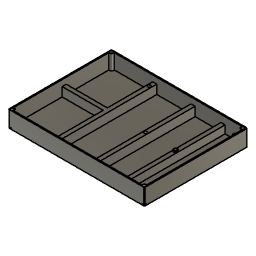
Housing_Base (Autodesk Fusion 360 design; units mm, degrees)
Autodesk Fusion 360 part; units mm, degrees
sketch "Sketch1" plane through (0, 0, 0) normal (0, 0, 1) x (1, 0, 0)
  line L0 (267, 172) -> (40, 172)
  line L1 (40, 172) -> (40, 0)
  line L2 (267, 0) -> (267, 172)
  circle A0 centre (114.1412, 160.8678) radius 2.55
  circle A1 centre (114.1412, 7.8678) radius 2.55
  circle A2 centre (257.1412, 7.8678) radius 2.55
  circle A3 centre (228.1412, 90.8678) radius 2.55
  circle A4 centre (178.1412, 90.8678) radius 2.55
  circle A5 centre (257.1412, 161.8678) radius 2.55
  line L3 (231.5912, 2) -> (231.5912, 170)
  line L4 (231.5912, 2) -> (231.5912, 170)
  line L5 (267, 172) -> (40, 172)
  line L6 (267, 2) -> (267, 172)
  line L7 (40, 0) -> (267, 0)
  line L8 (265, 6.0151) -> (265, 165.4022)
  line L9 (260.0451, 170) -> (231.5912, 170)
  arc A6 (42, 165.4407) -> (46.5116, 170) centre (43.2595, 168.7062) ccw
  arc A7 (42, 165.4407) -> (46.5116, 170) centre (43.2595, 168.7062) ccw
  arc A8 (46.8079, 2) -> (42, 6.1449) centre (43.4407, 2.9551) ccw
  line L10 (224.6912, 2) -> (224.6912, 87.4178)
  line L11 (224.6912, 94.3178) -> (224.6912, 170)
  line L12 (42, 165.4407) -> (42, 94.3178)
  line L13 (42, 87.4178) -> (42, 6.1449)
  line L14 (110.6912, 170) -> (46.5116, 170)
  line L15 (42, 94.3178) -> (110.6912, 94.3178)
  line L16 (117.5912, 2) -> (117.5912, 87.4178)
  line L17 (117.5912, 94.3178) -> (117.5912, 170)
  line L18 (109.8811, 164.7657) -> (109.8811, 94.3178) construction
  line L19 (109.8811, 87.4178) -> (109.8811, 4.2996) construction
  line L20 (42, 87.4178) -> (110.6912, 87.4178)
  line L21 (110.6912, 2) -> (110.6912, 87.4178)
  line L22 (110.6912, 94.3178) -> (110.6912, 170)
  line L23 (46.8079, 2) -> (110.6912, 2)
  arc A9 (260.0451, 170) -> (265, 165.4022) centre (263.1412, 168.3678) ccw
  arc A10 (265, 6.0151) -> (260.8505, 2) centre (263.9632, 2.9349) ccw
  line L24 (231.5912, 2) -> (260.8505, 2)
  circle A11 centre (257.1412, 7.8678) radius 4
  circle A12 centre (257.1412, 161.8678) radius 4
  circle A13 centre (228.1412, 90.8678) radius 3.45
  line L25 (117.5912, 94.3178) -> (117.5912, 87.4178)
  line L26 (224.6912, 170) -> (231.5912, 170)
  line L27 (224.6912, 2) -> (231.5912, 2)
  line L28 (224.6912, 94.3178) -> (224.6912, 87.4178)
  line L29 (40, 0) -> (267, 0)
  line L30 (267, 0) -> (267, 172)
  line L31 (267, 172) -> (40, 172)
  line L32 (40, 172) -> (40, 0)
  line L33 (174.6912, 2) -> (174.6912, 170)
  line L34 (181.5912, 2) -> (181.5912, 170)
  line L35 (224.6912, 170) -> (181.5912, 170)
  line L36 (174.6912, 170) -> (117.5912, 170)
  line L37 (117.5912, 2) -> (174.6912, 2)
  line L38 (181.5912, 2) -> (224.6912, 2)
  line L39 (42, 94.3178) -> (42, 87.4178)
  line L40 (110.6912, 170) -> (117.5912, 170)
  line L41 (110.6912, 2) -> (117.5912, 2)
  line L42 (174.6912, 2) -> (181.5912, 2)
  line L43 (174.6912, 170) -> (181.5912, 170)
  circle A14 centre (263.1412, 168.3678) radius 2.55
  circle A15 centre (263.9632, 2.9349) radius 2.55
  line L44 (263.9632, 2.9349) -> (260.7497, 2.9349)
  circle A16 centre (43.2595, 168.7062) radius 2.55
  circle A17 centre (43.4407, 2.9551) radius 2.55
  dimension "d7" = 5.1
  dimension "d8" = 5.1
  dimension "d9" = 5.1
  dimension "d10" = 5.1
  dimension "d11" = 5.1
  dimension "d12" = 5.1
  dimension "d20" = 7
  dimension "d21" = 7
  dimension "d26" = 7
  dimension "d28" = 6.5
  dimension "d29" = 8
  dimension "d30" = 8
  dimension "d37" = 6.9
  dimension "d51" = 6.9
  dimension "d90" = 5.1
  dimension "d91" = 5.1
  dimension "d92" = 5.1
  dimension "d93" = 5.1
  constraint vertical L18
  constraint coincident L3.start L23
  constraint coincident L1 L7.start
  constraint coincident L11.end L9
  constraint collinear L9 L35
  constraint collinear L23 L24
  constraint concentric A6 A7
  constraint perpendicular L10 L20
  constraint coincident L13.start L12
  constraint collinear L10 L11
  constraint collinear L12 L13
  constraint perpendicular L16 L35
  constraint coincident L16.start L23
  constraint collinear L14 L35
  constraint coincident L15.end L21
  constraint coincident L17.start L16
  constraint coincident L16.end L20
  constraint collinear L16 L17
  constraint coincident L15 L18.end
  constraint coincident L19.start L20
  constraint collinear L18 L19
  constraint collinear L21 L22
  constraint collinear L23 L37
  constraint concentric A2 A11
  constraint concentric A5 A12
  constraint concentric A3 A13
  constraint perpendicular L4 L26
  constraint perpendicular L4 L27
  constraint horizontal L29
  constraint vertical L30
  constraint horizontal L31
  constraint vertical L32
  constraint coincident L33.end L35
  constraint perpendicular L33 L35
  constraint collinear L35 L36
  constraint collinear L37 L38
  constraint perpendicular L20 L39
  constraint perpendicular L16 L41
  constraint concentric A9 A14
  constraint concentric A10 A15
  constraint coincident A10.centre A15.centre
  constraint horizontal L44
  constraint concentric A6 A16
  constraint concentric A8 A17
  measures "d7" diameter of A0
  measures "d8" diameter of A1
  measures "d9" diameter of A2
  measures "d10" diameter of A5
  measures "d11" diameter of A4
  measures "d12" diameter of A3
  measures "d20" diameter of A6
  measures "d21" diameter of A8
  measures "d26" diameter of A9
  measures "d28" diameter of A10
  measures "d29" diameter of A11
  measures "d30" diameter of A12
  measures "d37" diameter of A13
  measures "d90" diameter of A14
  measures "d91" diameter of A15
  measures "d92" diameter of A16
  measures "d93" diameter of A17
extrude "Extrude4" add sketch "Sketch1" along normal blind 27 contours L0 L1 L2 L5 L6 L7 L29 L30 L31 L32 | A14 | A15 | A16 | A17 makes body 1
extrude "Extrude5" add sketch "Sketch1" along normal blind 15 separate body contours L3 L4 L10 A13 L27 L28 | L3 L4 L11 A13 L26 L28 makes body 2 at (224.6912, 31.6226, 5)
extrude "Extrude9" add sketch "Sketch1" along normal blind 2 separate body contours A2 makes body 3
extrude "Extrude11" add sketch "Sketch1" along normal blind 2 separate body contours A5 makes body 4
extrude "Extrude12" add sketch "Sketch1" along normal blind 2 separate body contours A0 | A1 | A3 | A4 makes body 5 at (116.6123, 161.4971, 1.3333) makes body 6 at (230.6406, 90.3626, 1.3333) makes body 7 at (116.0946, 9.5069, 1.3333) makes body 8 at (180.6406, 90.3626, 1.3333)
extrude "Extrude13" add sketch "Sketch1" along normal blind 17 contours A13 bodies 2 6
extrude "Extrude14" add sketch "Sketch1" along normal blind 17 contours L33 L34 L42 L43 | L15 L16 L17 L20 L21 L22 L25 L39 L40 L41 | A11 | A12 bodies 1 3 4 5 7 8
extrude "Extrude15" add sketch "Sketch1" along normal blind 2 contours L3 L4 L8 L9 A9 A10 L24 | L10 L11 L28 L34 L35 L38 | L16 L17 L25 L33 L36 L37 | A8 L13 L20 L21 L23 | A6 A7 L12 L14 L15 L22 bodies 1 2 3 4
extrude "Extrude16" cut sketch "Sketch1" along normal blind 27 contours A14 | A15 | A16 | A17 bodies 1
extrude "Extrude17" add sketch "Sketch1" along normal blind 2 contours A14 | A15 | A16 | A17 bodies 1
fillet "Fillet1" radius 1 1 edges at (267, 0, 13.5) on bodies 1
fillet "Fillet1" radius 1 1 edges at (40, 0, 13.5) on bodies 1
fillet "Fillet1" radius 1 1 edges at (40, 172, 13.5) on bodies 1
fillet "Fillet2" radius 1 1 edges at (267, 172, 13.5) on bodies 1
